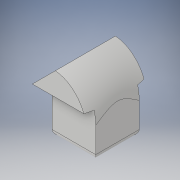
# Autodesk Inventor part: BUTTON_OUTSIDE
Saved by Autodesk Inventor 2019 (Build 230136000, 136)
## iProperties
Created: 2018-12-19
Part Number: BUTTON_OUTSIDE
Material: Типовые
Document SubType Name: Modeling
Designer: aldanstar
Density: 1 g/cm^3
Appearance: По умолчанию
Author: aldanstar
Autodesk Inventor part; units mm, degrees
ref_plane "YZ Plane" through (0, 0, 0) normal (1, 0, 0) x (0, 1, 0)
ref_plane "XZ Plane" through (0, 0, 0) normal (0, 1, 0) x (-1, 0, 0)
ref_plane "XY Plane" through (0, 0, 0) normal (0, 0, 1) x (1, 0, 0)
sketch "Эскиз1" plane through (0, 0, 0) normal (0, 1, 0) x (-1, 0, 0)
  line L0 (1.9, 1.9) -> (-1.9, 1.9)
  line L1 (-1.9, 1.9) -> (-1.9, -1.9)
  line L2 (-1.9, -1.9) -> (1.9, -1.9)
  line L3 (1.9, -1.9) -> (1.9, 1.9)
  line L4 (2.66, 0) -> (-2.66, 0) projected
  line L5 (0, -2.66) -> (0, 2.66) projected
  point P0 (0, 0)
  dimension "d0" = 3.8
  constraints: 8 end point, 2 parallel, 2 perpendicular, 1 horizontal, 2 other
  measures "d0" distance of L1.end L2.end
extrude "Выдавливание1" add sketch "Эскиз1" along normal blind 3.8
sketch "Эскиз2" plane through (0, 3.8, 0) normal (0, 1, 0) x (1, 0, 0)
  line L0 (-2.9, -2.625) -> (1.9, -2.625)
  line L1 (1.9, -2.625) -> (1.9, 2.625)
  line L2 (1.9, 2.625) -> (-2.9, 2.625)
  line L3 (-2.9, 2.625) -> (-2.9, -2.625)
  line L4 (1.9, -1.9) -> (1.9, 1.9) projected
  line L5 (-3.86, 0) -> (2.86, 0) projected
  point P0 (0, 0)
  dimension "d3" = 5.25
  dimension "d4" = 4.8
  constraints: 8 end point, 2 parallel, 1 collinear, 1 horizontal, 1 perpendicular, 1 other
  measures "d3" distance between parallel lines of L0 L2
  measures "d4" distance of L1.end L2.end
extrude "Выдавливание2" add sketch "Эскиз2" along normal blind 2
sketch "Эскиз5" plane through (1.9, 0, 1.9) normal (1, 0, 0) x (0, 0, -1)
  line L0 (4.525, 3.8) -> (4.525, 5.8) projected
  line L1 (-0.725, 5.8) -> (4.525, 5.8) projected
  line L2 (4.525, 5.8) -> (-0.725, 5.8)
  line L3 (-0.725, 3.8) -> (-0.725, 5.8) projected
  arc A0 (4.525, 5.8) -> (-0.725, 5.8) centre (1.9, 0.9668) ccw
  point P0 (1.9, 0)
  dimension "d10" = 5.5
  constraints: 2 end point, 2 point on circle, 1 centre point, 1 collinear
  measures "d10" radius of A0
chamfer "Фаска1" distance 2 angle 45 1 edges at (-2.9, 5.8, 0)
extrude "Выдавливание3" add sketch "Эскиз5" against normal up to surface surface through (-1.9, 4.8, -1.3125) normal (-0.7071068, 0.7071068, 0)
fillet "Сопряжение1" radius 3 1 edges at (1.9, 6.4668, 0)
fillet "Сопряжение2" radius 0.5 4 edges at (1.9, 0, 0) (0, 0, 1.9) (0, 0, -1.9) (-1.9, 0, 0)
